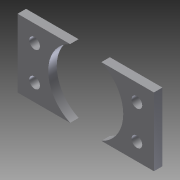
# Autodesk Inventor part: al_collar
Saved by Autodesk Inventor 2011 (Build 150239000, 239)
## iProperties
Created: 2012-06-13
Part Number: al_collar
Document SubType Name: Modeling
Designer: labuser
Density: 1 g/cm^3
Author: labuser
Autodesk Inventor part; units mm, degrees
ref_plane "YZ Plane" through (0, 0, 0) normal (1, 0, 0) x (0, 1, 0)
ref_plane "XZ Plane" through (0, 0, 0) normal (0, 1, 0) x (-1, 0, 0)
ref_plane "XY Plane" through (0, 0, 0) normal (0, 0, 1) x (1, 0, 0)
sketch "Sketch1" plane through (0, 0, 0) normal (0, 0, 1) x (1, 0, 0)
  line L0 (-12.7, -6.35) -> (12.7, -6.35)
  line L1 (12.7, -6.35) -> (12.7, 6.35)
  line L2 (12.7, 6.35) -> (-12.7, 6.35)
  line L3 (-12.7, 6.35) -> (-12.7, -6.35)
  point P0 (0, 0)
  dimension "d0" = 25.4
  dimension "d1" = 12.7
  constraints: 8 end point, 2 parallel, 1 horizontal, 1 perpendicular
  measures "d0" distance of L2.end L1.end
  measures "d1" distance of L1.end L0.end
extrude "Extrusion1" add sketch "Sketch1" along normal blind 1.5875
sketch "Sketch2" plane through (0, 0, 1.5875) normal (0, 0, 1) x (1, 0, 0)
  circle A0 centre (0, 0) radius 6.985
  dimension "d4" = 13.97
  constraints: 1 centre point, 1 coincident
  measures "d4" diameter of A0
extrude "Extrusion2" cut sketch "Sketch2" against normal through all
sketch "Sketch6" plane through (0, 0, 1.5875) normal (0, 0, 1) x (1, 0, 0)
  point P0 (0, 0)
  point P1 (-9.525, -3.175)
  point P2 (-9.525, 3.175)
  point P3 (9.525, 3.175)
  point P4 (9.525, -3.175)
hole "Hole3" at (-9.525, -3.175, 1.5875) at (-9.525, 3.175, 1.5875) at (9.525, 3.175, 1.5875) at (9.525, -3.175, 1.5875) direction (0, 0, -1) diameter 2 depth 25.4 tip angle 118
body "Solid1"
